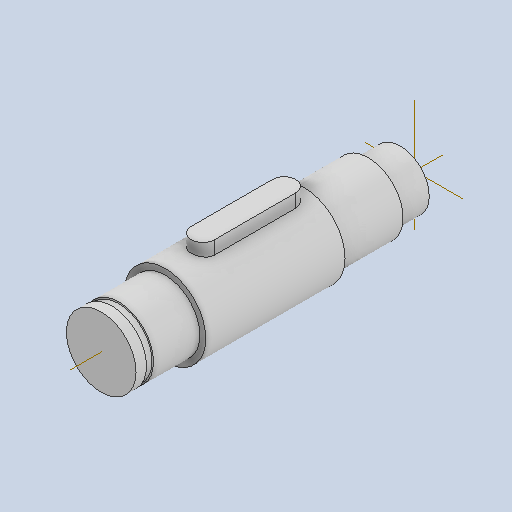
# Autodesk Inventor part: shatft extension
Saved by Autodesk Inventor 2025.2 (Build 292293000, 293)
## iProperties
Created: 2025-02-28
Part Number: shatft extension
Material: Generic
Document SubType Name: Modeling
Designer: zeyad
Density: 1 g/cm^3
Appearance: Default
Author: zeyad
Autodesk Inventor part; units mm, degrees
sketch "Sketch1" plane through (0, 0, 0) normal (0, 0, 1) x (1, 0, 0)
  arc A0 (-1.5, -1.3229) -> (-1.5, 1.3229) centre (0, 0) ccw
  line L0 (-1.5, 1.3229) -> (-1.5, -1.3229)
  circle A1 centre (0, 0) radius 5
  dimension "d0" = 4
  dimension "d2" = 10
  constraints: 2 centre point, 2 coincident, 2 end point, 2 point on circle, 1 vertical
  measures "d0" diameter of A0
  measures "d2" diameter of A1
extrude "Extrusion1" add sketch "Sketch1" along normal blind 8
sketch "Sketch2" plane through (0, 0, 8) normal (0, 0, 1) x (1, 0, 0)
  point P0 (0, 0)
sketch "Sketch3" plane through (0, 0, 8) normal (0, 0, 1) x (1, 0, 0)
  circle A0 centre (0, 0) radius 7
  dimension "d5" = 14
  constraints: 1 centre point, 1 coincident
  measures "d5" diameter of A0
extrude "Extrusion2" add sketch "Sketch3" along normal blind 35
ref_plane "Work Plane1" through (0, 9, 0) normal (0, 1, 0) x (-1, 0, 0)
sketch "Sketch4" plane through (0, 9, 0) normal (0, 1, 0) x (-1, 0, 0)
  line L0 (0, 20.5) -> (0, 20.5)
  line L1 (-2, 22.5) -> (-2, 36.5)
  line L2 (0, 38.5) -> (0, 38.5)
  line L3 (2, 36.5) -> (2, 22.5)
  line L4 (0, -7.7828) -> (0, 46.6971) projected
  line L5 (7, 8) -> (-7, 8) projected
  arc A0 (0, 20.5) -> (2, 22.5) centre (0, 22.5) ccw
  arc A1 (-2, 22.5) -> (0, 20.5) centre (0, 22.5) ccw
  arc A2 (2, 36.5) -> (0, 38.5) centre (0, 36.5) ccw
  arc A3 (0, 38.5) -> (-2, 36.5) centre (0, 36.5) ccw
  line L6 (4.0307, 31) -> (-5.3749, 31) construction
  point P0 (0, 0)
  point P1 (-2, 38.5)
  point P2 (-2, 20.5)
  point P3 (2, 38.5)
  point P4 (0, 38.5)
  point P5 (0, 20.5)
  point P6 (0, 38.5)
  point P7 (0, 20.5)
  point P8 (0, 20.5)
  point P9 (0, 38.5)
  dimension "d9" = 18
  dimension "d10" = 4
  dimension "d11" = 12.5
  dimension "d12" = 2
  constraints: 10 end point, 8 point on circle, 8 tangent, 6 point on line, 4 centre point, 3 equal radius, 2 horizontal, 2 parallel, 1 perpendicular, 1 other
  measures "d9" distance of point (-2, 20.5) point (-2, 38.5)
  measures "d10" distance of point (-2, 38.5) point (2, 38.5)
  measures "d11" distance between parallel lines of L0 L5
  measures "d12" radius of A0
extrude "Extrusion3" add sketch "Sketch4" against normal up to surface
sketch "Sketch5" plane through (0, 0, 8) normal (0, 0, -1) x (-1, 0, 0)
  circle A0 centre (0, 0) radius 6
  circle A1 centre (0, 0) radius 7
  dimension "d15" = 12
  constraints: 2 centre point, 2 coincident
  measures "d15" diameter of A0
extrude "Extrusion4" cut sketch "Sketch5" against normal blind 11
sketch "Sketch6" plane through (0, 0, 43) normal (0, 0, 1) x (1, 0, 0)
  arc A0 (-1.5, -1.3229) -> (-1.5, 1.3229) centre (0, 0) ccw projected
  circle A1 centre (0, 0) radius 6
  dimension "d18" = 12
  constraints: 1 centre point, 1 coincident
  measures "d18" diameter of A1
extrude "Extrusion5" add sketch "Sketch6" along normal blind 11
ref_plane "Work Plane2" through (0, 0, 11) normal (0, 0, -1) x (-1, 0, 0)
ref_plane "Work Plane3" through (0, 0, 51) normal (0, 0, 1) x (1, 0, 0)
sketch "Sketch8" plane through (0, 0, 51) normal (0, 0, 1) x (1, 0, 0)
  circle A0 centre (0, 0) radius 5.75
  arc A1 (-1.5, -1.3229) -> (-1.5, 1.3229) centre (0, 0) ccw projected
  circle A2 centre (0, 0) radius 6
  dimension "d27" = 11.5
  dimension "d28" = 12
  constraints: 2 centre point, 2 coincident
  measures "d27" diameter of A0
  measures "d28" diameter of A2
extrude "Extrusion7" cut sketch "Sketch8" along normal blind 1.2
sketch "Sketch9" plane through (0, 0, 0) normal (0, 0, -1) x (-1, 0, 0)
  circle A0 centre (0, 0) radius 5 projected
  line L0 (1.5, -1.3229) -> (1.5, 1.3229) projected
  arc A1 (1.5, 1.3229) -> (1.5, -1.3229) centre (0, 0) ccw projected
extrude "Extrusion8" cut sketch "Sketch9" against normal blind 2.5
sketch "Sketch10" plane through (0, 0, 8) normal (0, 0, -1) x (-1, 0, 0)
  arc A0 (1.5, 1.3229) -> (1.5, -1.3229) centre (0, 0) ccw projected
  line L0 (1.5, -1.3229) -> (1.5, 1.3229) projected
extrude "Extrusion9" cut sketch "Sketch10" against normal blind 2.7
sketch "Sketch11" plane through (0, 0, 8) normal (0, 0, -1) x (-1, 0, 0)
  line L0 (1.5, 1.3229) -> (1.5, -1.3229) projected
  arc A0 (1.5, 1.3229) -> (1.5, -1.3229) centre (0, 0) ccw projected
extrude "Extrusion10" add sketch "Sketch11" along normal up to surface (5.5 mm away)
sketch "Sketch12" plane through (0, 0, 2.5) normal (0, 0, -1) x (-1, 0, 0)
  circle A0 centre (0, 0) radius 1.5 projected
  line L0 (-2.5408, -1.5951) -> (-2.4576, 1.7205) projected
  arc A1 (-2.5408, -1.5951) -> (-2.4576, 1.7205) centre (0, 0) ccw projected
  point P0 (0, 0)
extrude "Extrusion11" cut sketch "Sketch12" against normal blind 12 contours A0 | L0 A1
body "Solid1"
